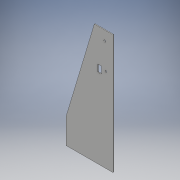
# Autodesk Inventor part: Part2
Saved by Autodesk Inventor 2018 (Build 220112000, 112)
## iProperties
Created: 2018-06-07
Part Number: Part2
Material: 一般
Document SubType Name: Modeling
Designer: ku_sk
Density: 1 g/cm^3
Appearance: 既定
Author: ku_sk
Autodesk Inventor part; units mm, degrees
ref_plane "YZ Plane" through (0, 0, 0) normal (1, 0, 0) x (0, 1, 0)
ref_plane "XZ Plane" through (0, 0, 0) normal (0, 1, 0) x (-1, 0, 0)
ref_plane "XY Plane" through (0, 0, 0) normal (0, 0, 1) x (1, 0, 0)
sketch "スケッチ1" plane through (0, 0, 0) normal (0, 1, 0) x (-1, 0, 0)
  line L0 (0, 254.5) -> (0, -254.5)
  line L1 (0, -254.5) -> (200, -254.5)
  line L2 (200, -254.5) -> (200, -145.5)
  line L3 (200, -145.5) -> (80, 254.5)
  line L4 (80, 254.5) -> (0, 254.5)
  point P0 (0, 0)
  point P1 (0, 0)
  dimension "d0" = 509
  dimension "d1" = 200
  dimension "d2" = 109
  dimension "d3" = 80
  constraints: 10 end point, 2 perpendicular, 1 coincident, 1 midpoint, 1 parallel, 1 vertical
  measures "d0" distance of L0.start L0.end
  measures "d1" distance of L0.end L1.end
  measures "d2" distance of L1.end L2.end
  measures "d3" distance of L3.end L0.start
extrude "押し出し1" add sketch "スケッチ1" along normal blind 3
sketch "スケッチ2" plane through (0, 0, 0) normal (0, -1, 0) x (1, 0, 0)
  circle A0 centre (-35.142, 214.391) radius 4.25
  circle A1 centre (-30.426, 103.793) radius 4.25
  line L0 (-65, 84.5) -> (-50, 84.5)
  line L1 (-50, 84.5) -> (-50, 114.5)
  line L2 (-50, 114.5) -> (-65, 114.5)
  line L3 (-65, 114.5) -> (-65, 84.5)
  line L4 (-80, 254.5) -> (0, 254.5) projected
  line L5 (0, 254.5) -> (0, -254.5) projected
  point P0 (0, 0)
  dimension "d6" = 15
  dimension "d7" = 30
  dimension "d8" = 8.5
  dimension "d9" = 8.5
  dimension "d10" = 40.109
  dimension "d11" = 35.142
  dimension "d12" = 150.707
  dimension "d13" = 30.426
  dimension "d14" = 140
  dimension "d15" = 50
  constraints: 8 end point, 2 centre point, 2 parallel, 1 horizontal, 1 perpendicular
  measures "d6" distance of L1.end L2.end
  measures "d7" distance of L0.end L1.end
  measures "d8" diameter of A1
  measures "d9" diameter of A0
  measures "d10" distance from line of L4 A0.centre
  measures "d11" distance from line of A0.centre L5
  measures "d12" distance from line of L4 A1.centre
  measures "d13" distance from line of L5 A1.centre
  measures "d14" distance between parallel lines of L4 L2
  measures "d15" distance between parallel lines of L5 L1
extrude "押し出し2" cut sketch "スケッチ2" against normal blind 3
fillet "フィレット1" radius 1 9 edges at (-80, 1.5, 254.5) (0, 1.5, 254.5) (-200, 1.5, -145.5) (-200, 1.5, -254.5) (0, 1.5, -254.5) (-50, 1.5, 84.5) (-50, 1.5, 114.5) (-65, 1.5, 114.5) (-65, 1.5, 84.5)
